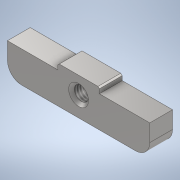
# Autodesk Inventor part: 0 零件
Saved by Autodesk Inventor 2020 (Build 240168000, 168)
## iProperties
Created: 2020-11-03
Part Number: 0 零件
Material: 不鏽鋼
Document SubType Name: Sheet Metal
Designer: p2013
Density: 8 g/cm^3
Appearance: 不鏽鋼 - 疏刷(1)
Sheet Metal Rule: 預設 mm (_M)
Author: p2013
Autodesk Inventor part; units mm, degrees
ref_plane "YZ Plane" through (0, 0, 0) normal (1, 0, 0) x (0, 1, 0)
ref_plane "XZ Plane" through (0, 0, 0) normal (0, 1, 0) x (-1, 0, 0)
ref_plane "XY Plane" through (0, 0, 0) normal (0, 0, 1) x (1, 0, 0)
sketch "草圖1" plane through (0, 0, 0) normal (0, 0, 1) x (1, 0, 0)
  line L0 (0, 0) -> (-25.6572, 0) construction
  line L1 (0, 0) -> (0, 25.6407) construction
  line L2 (-20, -5.5) -> (-8.1185, -5.5)
  line L3 (25, -0.5) -> (25, 5.5)
  line L4 (25, 5.5) -> (-25, 5.5)
  line L5 (-25, 5.5) -> (-25, -0.5)
  line L6 (-25, -5.5) -> (25, 5.5) construction
  line L7 (25, -5.5) -> (-25, 5.5) construction
  arc A0 (20, -5.5) -> (25, -0.5) centre (20, -0.5) ccw
  arc A1 (-25, -0.5) -> (-20, -5.5) centre (-20, -0.5) ccw
  line L8 (-8.1185, -5.5) -> (20, -5.5)
  line L9 (7.3, 5.5) -> (7.3, 7)
  line L10 (6.8, 7.5) -> (-6.8, 7.5)
  line L11 (-7.3, 7) -> (-7.3, 5.5)
  circle A2 centre (0, 1.5) radius 2.5
  line L12 (-7.3, 7) -> (-6.8, 7.5)
  line L13 (6.8, 7.5) -> (7.3, 7)
  point P0 (7.3, 7.5)
  point P1 (-7.3, 7.5)
  dimension "d0" = 50
  dimension "d4" = 5
  dimension "d13" = 2
  dimension "d14" = 14.6
  dimension "d15" = 5
  dimension "d20" = 0.5
  dimension "d21" = 0.5
  dimension "d22" = 0.5
  dimension "d23" = 0.5
  dimension "d27" = 11
  dimension "d28" = 4
  constraints: 28 end point, 15 point on line, 6 tangent, 4 parallel, 4 point on circle, 3 centre point, 3 horizontal, 2 midpoint, 2 perpendicular, 2 vertical, 1 equal radius, 1 other
  measures "d0" distance between parallel lines of L3 L5
  measures "d4" radius of A0
  measures "d13" distance between parallel lines of L4 L10
  measures "d14" distance between parallel lines of L11 L9
  measures "d15" diameter of A2
  measures "d20" distance of L11.start point (-7.3, 7.5)
  measures "d21" distance of L10.end point (-7.3, 7.5)
  measures "d22" distance of L10.start point (7.3, 7.5)
  measures "d23" distance of L9.end point (7.3, 7.5)
  measures "d27" distance between parallel lines of L4 L8
  measures "d28" distance from line of A2.centre L4
extrude "擠出1" add sketch "草圖1" along normal mid plane 8
thread "螺紋1" size "M6x1" class "6H" standard "ANSI Metric M Profile" full length
chamfer "倒角1" distance 1 angle 45 1 edges at (-2.5, 1.5, 4)
equation "\"d21\" = d20"
equation "\"d22\" = d20"
equation "\"d23\" = d22"
equation "\"折彎半徑\" = 厚度"
equation "\"折彎離隙寬度\" = 厚度"
equation "\"折彎離隙深度\" = 0.5 * 厚度"
equation "\"轉角離隙大小\" = 4 * 厚度"
equation "\"最小剩餘\" = 2 * 厚度"
equation "\"轉移半徑\" = 折彎半徑"
equation "\"Jacobi半徑大小\" = 折彎半徑"
equation "\"間隙大小\" = 厚度"
equation "\"厚度\" = 8"
